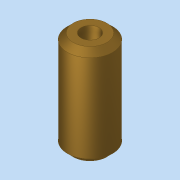
# Autodesk Inventor part: MotorShaftCoupler
Saved by Autodesk Inventor 2017 (Build 210142000, 142)
## iProperties
Created: 2016-10-13
Part Number: MotorShaftCoupler
Material: Generic
Document SubType Name: Modeling
Designer: techn
Density: 1 g/cm^3
Appearance: Brass - Satin
Author: techn
Autodesk Inventor part; units mm, degrees
ref_plane "YZ Plane" through (0, 0, 0) normal (1, 0, 0) x (0, 1, 0)
ref_plane "XZ Plane" through (0, 0, 0) normal (0, 1, 0) x (-1, 0, 0)
ref_plane "XY Plane" through (0, 0, 0) normal (0, 0, 1) x (1, 0, 0)
sketch "Sketch1" plane through (0, 0, 0) normal (0, 0, 1) x (1, 0, 0)
  line L0 (0, 0) -> (5, 0)
  line L1 (5, 0) -> (5, 22)
  line L2 (5, 22) -> (0, 22)
  line L3 (0, 0) -> (1.585, 0)
  line L4 (1.585, 0) -> (1.585, 11)
  line L5 (0, 22) -> (2, 22)
  line L6 (2, 22) -> (2, 11)
  line L7 (2, 11) -> (1.585, 11)
  circle A0 centre (0, 17) radius 1.5
  circle A1 centre (0, 5) radius 1.5
  line L8 (0, 0) -> (0, -2.0166)
  dimension "d0" = 5
  dimension "d1" = 22
  dimension "d2" = 1.585
  dimension "d3" = 2
  dimension "d4" = 3
  dimension "d5" = 3
  dimension "d6" = 5
  dimension "d7" = 5
  constraints: 18 end point, 5 perpendicular, 2 centre point, 2 point on line, 1 horizontal, 1 vertical
  measures "d0" distance of L0.start L0.end
  measures "d1" distance of L0.end L1.end
  measures "d2" distance of L0.start L3.end
  measures "d3" distance of L2.end L5.end
  measures "d4" diameter of A0
  measures "d5" diameter of A1
  measures "d6" distance from line of L2 A0.centre
  measures "d7" distance from line of L0 A1.centre
revolve "Revolution1" add sketch "Sketch1" angle 360 about axis through (0, 0, 0) along (0, -1, 0) contours L4 L7 L6 L2 L1 L0
extrude "Extrusion1" cut sketch "Sketch1" against normal blind 25.4 contours A0 | A1
chamfer "Chamfer1" distance 1.27 angle 45 2 edges at (-5, 22, 0) (-5, 0, 0)
body "Solid1"
